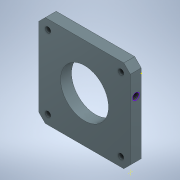
# Autodesk Inventor part: attachment motor
Saved by Autodesk Inventor 2021.2 (Build 252289000, 289)
## iProperties
Created: 2024-04-19
Part Number: attachment motor
Material: Lead
Document SubType Name: Modeling
Designer: cioba
Density: 11.34 g/cm^3
Appearance: Lead
Author: cioba
Autodesk Inventor part; units mm, degrees
ref_plane "YZ Plane" through (0, 0, 0) normal (1, 0, 0) x (0, 1, 0)
ref_plane "XZ Plane" through (0, 0, 0) normal (0, 1, 0) x (-1, 0, 0)
ref_plane "XY Plane" through (0, 0, 0) normal (0, 0, 1) x (1, 0, 0)
sketch "Sketch1" plane through (0, 0, 0) normal (0, 0, 1) x (1, 0, 0)
  line L0 (-3.9016, 5.1111) -> (32.0984, 5.1111)
  line L1 (35.0984, 2.1111) -> (35.0984, -33.8889)
  line L2 (32.0984, -36.8889) -> (-3.9016, -36.8889)
  line L3 (-6.9016, -33.8889) -> (-6.9016, 2.1111)
  circle A0 centre (14.0984, -15.8889) radius 11
  line L4 (35.0984, 2.1111) -> (32.0984, 5.1111)
  line L5 (-6.9016, 2.1111) -> (-3.9016, 5.1111)
  line L6 (-6.9016, -33.8889) -> (-3.9016, -36.8889)
  line L7 (35.0984, -33.8889) -> (32.0984, -36.8889)
  circle A1 centre (30.8484, -32.6389) radius 1.25
  circle A2 centre (-2.6516, -32.6389) radius 1.25
  circle A3 centre (-2.6516, 0.8611) radius 1.25
  circle A4 centre (30.8484, 0.8611) radius 1.25
  point P0 (0, 0)
  constraints: 16 end point, 5 centre point, 2 parallel, 1 horizontal, 1 perpendicular
extrude "Extrusion8" add sketch "Sketch1" along normal blind 5
sketch "Sketch2" plane through (35.0984, -33.8889, 0) normal (1, 0, 0) x (0, 0, -1)
  circle A0 centre (-2.5, 26) radius 1.5
  point P0 (0, 33.8889)
  point P1 (-5, -3)
  constraints: 1 centre point
hole "Hole1" at (35.0984, -7.8889, 2.5) direction (-1, 0, 0) diameter 3 depth 5 tip angle 118
sketch "Sketch3" plane through (-6.9016, -33.8889, 0) normal (-1, 0, 0) x (0, 0, 1)
  circle A0 centre (2.5, 26) radius 1.5 projected
  circle A1 centre (2.5, 26) radius 1.5
  point P0 (0, 33.8889)
  constraints: 1 centre point, 1 coincident
hole "Hole3" at (-6.9016, -7.8889, 2.5) direction (1, 0, 0) diameter 3 depth 5 tip angle 118
thread "Thread1" size "M3x0.5" class "6H" standard "ANSI Metric M Profile" full length
thread "Thread2" size "M3x0.5" class "6H" standard "ANSI Metric M Profile" full length
body "Solid1"
